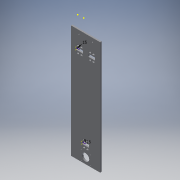
# Autodesk Inventor part: XCartFloor
Saved by Autodesk Inventor 2019 (Build 230136000, 136)
## iProperties
Created: 2019-08-19
Part Number: XCartFloor
Material: Generic
Document SubType Name: Modeling
Designer: Bruno
Density: 1 g/cm^3
Appearance: Default
Author: Bruno
Autodesk Inventor part; units mm, degrees
ref_plane "YZ Plane" through (0, 0, 0) normal (1, 0, 0) x (0, 1, 0)
ref_plane "XZ Plane" through (0, 0, 0) normal (0, 1, 0) x (-1, 0, 0)
ref_plane "XY Plane" through (0, 0, 0) normal (0, 0, 1) x (1, 0, 0)
sketch "Sketch1" plane through (0, 0, 0) normal (0, 0, 1) x (1, 0, 0)
  line L0 (100, -38.5222) -> (0, -38.5222)
  line L1 (0, -38.5222) -> (0, -426.5222)
  line L2 (0, -426.5222) -> (100, -426.5222)
  line L3 (100, -426.5222) -> (100, -38.5222)
  line L4 (82.6667, -93.1222) -> (58.6667, -93.1222)
  line L5 (58.6667, -93.1222) -> (58.6667, -101.9222)
  line L6 (58.6667, -101.9222) -> (82.6667, -101.9222)
  line L7 (82.6667, -101.9222) -> (82.6667, -93.1222)
  line L8 (41.3333, -93.1222) -> (17.3333, -93.1222)
  line L9 (17.3333, -93.1222) -> (17.3333, -101.9222)
  line L10 (17.3333, -101.9222) -> (41.3333, -101.9222)
  line L11 (41.3333, -101.9222) -> (41.3333, -93.1222)
  line L12 (38, -363.1222) -> (62, -363.1222)
  line L13 (62, -363.1222) -> (62, -371.9222)
  line L14 (62, -371.9222) -> (38, -371.9222)
  line L15 (38, -371.9222) -> (38, -363.1222)
  line L16 (173.8639, -93.5222) -> (-221.1361, -93.5222)
  line L17 (173.8639, -101.5222) -> (-221.1361, -101.5222)
  line L18 (173.8639, -371.5222) -> (-221.1361, -371.5222)
  line L19 (173.8639, -363.5222) -> (-221.1361, -363.5222)
  line L20 (34.8712, -93.1222) -> (34.8712, -93.5222) construction
  line L21 (34.8712, -101.5222) -> (34.8712, -101.9222) construction
  line L22 (82.6667, -93.1222) -> (100, -93.1222) construction
  line L23 (58.6667, -93.1222) -> (41.3333, -93.1222) construction
  line L24 (17.3333, -93.1222) -> (0, -93.1222) construction
  line L25 (10.9151, -363.1222) -> (10.9151, -363.5222) construction
  line L26 (10.9151, -371.5222) -> (10.9151, -371.9222) construction
  line L27 (38, -363.1222) -> (0, -363.1222) construction
  line L28 (62, -363.1222) -> (100, -363.1222) construction
  line L29 (0, 0) -> (0, -9.7735) construction
  circle A0 centre (65.5, -390.5222) radius 1.625
  circle A1 centre (65.5, -421.5222) radius 1.625
  circle A2 centre (34.5, -421.5222) radius 1.625
  circle A3 centre (34.5, -390.5222) radius 1.625
  line L30 (65.5, -390.5222) -> (34.5, -390.5222) construction
  line L31 (34.5, -390.5222) -> (34.5, -421.5222) construction
  line L32 (34.5, -421.5222) -> (65.5, -421.5222) construction
  line L33 (65.5, -421.5222) -> (65.5, -390.5222) construction
  line L34 (34.5, -390.5222) -> (0, -390.5222) construction
  line L35 (65.5, -390.5222) -> (100, -390.5222) construction
  circle A4 centre (50, -406.0222) radius 12.5
  line L36 (50, -390.5222) -> (50, -406.0222) construction
  line L37 (50, -406.0222) -> (65.5, -406.0222) construction
  line L38 (72.1667, -84.1222) -> (80.1667, -84.1222)
  line L39 (80.1667, -84.1222) -> (80.1667, -88.1222)
  line L40 (80.1667, -88.1222) -> (72.1667, -88.1222)
  line L41 (72.1667, -88.1222) -> (72.1667, -84.1222)
  line L42 (80.1667, -88.1222) -> (82.6667, -88.1222) construction
  line L43 (82.6667, -88.1222) -> (82.6667, -93.1222) construction
  line L44 (69.1667, -84.1222) -> (61.1667, -84.1222)
  line L45 (61.1667, -84.1222) -> (61.1667, -88.1222)
  line L46 (61.1667, -88.1222) -> (69.1667, -88.1222)
  line L47 (69.1667, -88.1222) -> (69.1667, -84.1222)
  line L48 (58.6667, -93.1222) -> (58.6667, -88.1222) construction
  line L49 (58.6667, -88.1222) -> (61.1667, -88.1222) construction
  line L50 (72.1667, -106.9222) -> (80.1667, -106.9222)
  line L51 (80.1667, -106.9222) -> (80.1667, -110.9222)
  line L52 (80.1667, -110.9222) -> (72.1667, -110.9222)
  line L53 (72.1667, -110.9222) -> (72.1667, -106.9222)
  line L54 (80.1667, -106.9222) -> (80.1667, -101.9222) construction
  line L55 (69.1667, -106.9222) -> (61.1667, -106.9222)
  line L56 (61.1667, -106.9222) -> (61.1667, -110.9222)
  line L57 (61.1667, -110.9222) -> (69.1667, -110.9222)
  line L58 (69.1667, -110.9222) -> (69.1667, -106.9222)
  line L59 (38.8333, -84.1222) -> (30.8333, -84.1222)
  line L60 (30.8333, -84.1222) -> (30.8333, -88.1222)
  line L61 (30.8333, -88.1222) -> (38.8333, -88.1222)
  line L62 (38.8333, -88.1222) -> (38.8333, -84.1222)
  line L63 (27.8333, -84.1222) -> (19.8333, -84.1222)
  line L64 (19.8333, -84.1222) -> (19.8333, -88.1222)
  line L65 (19.8333, -88.1222) -> (27.8333, -88.1222)
  line L66 (27.8333, -88.1222) -> (27.8333, -84.1222)
  line L67 (30.8333, -106.9222) -> (38.8333, -106.9222)
  line L68 (38.8333, -106.9222) -> (38.8333, -110.9222)
  line L69 (38.8333, -110.9222) -> (30.8333, -110.9222)
  line L70 (30.8333, -110.9222) -> (30.8333, -106.9222)
  line L71 (27.8333, -106.9222) -> (19.8333, -106.9222)
  line L72 (19.8333, -106.9222) -> (19.8333, -110.9222)
  line L73 (19.8333, -110.9222) -> (27.8333, -110.9222)
  line L74 (27.8333, -110.9222) -> (27.8333, -106.9222)
  line L75 (41.3333, -93.1222) -> (41.3333, -88.1222) construction
  line L76 (41.3333, -88.1222) -> (38.8333, -88.1222) construction
  line L77 (17.3333, -93.1222) -> (17.3333, -88.1222) construction
  line L78 (17.3333, -88.1222) -> (19.8333, -88.1222) construction
  line L79 (51.5, -354.1222) -> (59.5, -354.1222)
  line L80 (59.5, -354.1222) -> (59.5, -358.1222)
  line L81 (59.5, -358.1222) -> (51.5, -358.1222)
  line L82 (51.5, -358.1222) -> (51.5, -354.1222)
  line L83 (48.5, -354.1222) -> (40.5, -354.1222)
  line L84 (40.5, -354.1222) -> (40.5, -358.1222)
  line L85 (40.5, -358.1222) -> (48.5, -358.1222)
  line L86 (48.5, -358.1222) -> (48.5, -354.1222)
  line L87 (51.5, -376.9222) -> (59.5, -376.9222)
  line L88 (59.5, -376.9222) -> (59.5, -380.9222)
  line L89 (59.5, -380.9222) -> (51.5, -380.9222)
  line L90 (51.5, -380.9222) -> (51.5, -376.9222)
  line L91 (48.5, -376.9222) -> (40.5, -376.9222)
  line L92 (40.5, -376.9222) -> (40.5, -380.9222)
  line L93 (40.5, -380.9222) -> (48.5, -380.9222)
  line L94 (48.5, -380.9222) -> (48.5, -376.9222)
  line L95 (59.5, -358.1222) -> (62, -358.1222) construction
  line L96 (62, -358.1222) -> (62, -363.1222) construction
  line L97 (38, -363.1222) -> (38, -358.1222) construction
  line L98 (38, -358.1222) -> (40.5, -358.1222) construction
  line L99 (59.5, -376.9222) -> (59.5, -371.9222) construction
  circle A5 centre (73.5, -50.5222) radius 2.125
  circle A6 centre (26.5, -50.5222) radius 2.125
  line L100 (73.5, -50.5222) -> (100, -50.5222) construction
  line L101 (26.5, -50.5222) -> (0, -50.5222) construction
  line L102 (96.5, -57.5222) -> (88.5, -57.5222) projected
  line L103 (11.5, -57.5222) -> (3.5, -57.5222) projected
  line L104 (8, -43.5222) -> (8, -57.5222) projected
  line L105 (7, -57.5222) -> (7, -43.5222) projected
  line L106 (93, -43.5222) -> (93, -57.5222) projected
  line L107 (92, -57.5222) -> (92, -43.5222) projected
  line L108 (7.5, -57.5222) -> (7.5, -426.5222) construction
  line L109 (92.5, -57.5222) -> (92.5, -426.5222) construction
  circle A7 centre (92.5, -419.5222) radius 2.125
  circle A8 centre (92.5, -392.5222) radius 2.125
  circle A9 centre (7.5, -419.5222) radius 2.125
  circle A10 centre (7.5, -392.5222) radius 2.125
  line L110 (92.5, -419.5222) -> (7.5, -419.5222) construction
  line L111 (92.5, -392.5222) -> (7.5, -392.5222) construction
  dimension "d1" = 24
  dimension "d2" = 8.8
  dimension "d3" = 100
  dimension "d9" = 55
  dimension "d10" = 55
  dimension "d11" = 3.25
  dimension "d12" = 31
  dimension "d13" = 5
  dimension "d14" = 25
  dimension "d15" = 4
  dimension "d16" = 8
  dimension "d17" = 5
  dimension "d18" = 2.5
  dimension "d19" = 4.25
  dimension "d20" = 4.25
  dimension "d21" = 47
  dimension "d22" = 12
  dimension "d23" = 4.25
  dimension "d24" = 4.25
  dimension "d25" = 27
  dimension "d26" = 7
  dimension "d27" = 4.25
  dimension "d28" = 4.25
  constraints: 212 end point, 48 point on line, 38 equal length, 33 parallel, 30 perpendicular, 24 horizontal, 11 centre point, 9 vertical, 8 collinear, 4 midpoint, 3 equal radius, 8 other
  measures "d1" distance of L5.end L6.end
  measures "d2" distance of L4.end L5.end
  measures "d3" distance of L0.start L0.end
  measures "d9" distance between parallel lines of L0 L16
  measures "d10" distance between parallel lines of L2 L18
  measures "d11" diameter of A0
  measures "d12" distance of L32.end L30.start
  measures "d13" distance between parallel lines of L2 L32
  measures "d14" diameter of A4
  measures "d15" distance of L38.end L39.end
  measures "d16" distance of L38.start L38.end
  measures "d17" distance of L42.end L4.start
  measures "d18" distance of L39.end L42.end
  measures "d19" diameter of A5
  measures "d20" diameter of A6
  measures "d21" distance of L101.start L100.start
  measures "d22" distance between parallel lines of L0 L100
  measures "d23" diameter of A7
  measures "d24" diameter of A8
  measures "d25" distance of L110.start L111.start
  measures "d26" distance from line of L2 L110.start
  measures "d27" diameter of A9
  measures "d28" diameter of A10
extrude "Extrusion1" add sketch "Sketch1" along normal blind 5 contours L3 L16 L7 L4 L5 L11 L8 L9 L1 L0 | L3 L17 L7 L16 | L16 L9 L17 L1 | L3 L19 L13 L12 L15 L1 L17 L9 L10 L11 L5 L6 L7 | L3 L18 L13 L19 | L5 L17 L11 L16 | L19 L15 L18 L1 | L3 L2 L1 L18 L15 L14 L13
sketch "Sketch2" plane through (17.3333, -101.9222, 0) normal (1, 0, 0) x (0, 0, -1)
  circle A0 centre (6.0737, 4.4) radius 7.5
  point P0 (0, 101.9222)
  point P1 (0, 8.8)
  point P2 (0, 0)
  dimension "d6" = 15
  constraints: 2 point on circle, 1 centre point
  measures "d6" diameter of A0
sketch "Sketch3" plane through (38, -371.9222, 0) normal (1, 0, 0) x (0, 0, -1)
  circle A0 centre (6.0737, 4.4) radius 7.5
  point P0 (0, 371.9222)
  point P1 (0, 8.8)
  point P2 (0, 0)
  dimension "d8" = 15
  constraints: 2 point on circle, 1 centre point
  measures "d8" diameter of A0
body "Solid1"
